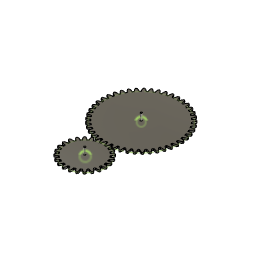
Task 5 v1 (Autodesk Fusion 360 design; units mm, degrees)
description: Spur Gear; Module: 12.700000; Num Teeth: 24; Pressure Angle: 20.000000; Backlash: 0.00 mm
description: Spur Gear; Module: 12.7; Num Teeth: 45; Pressure Angle: 20.0; Backlash: 0.00 mm
Autodesk Fusion 360 part; units mm, degrees
(part 1 of 8)
sketch "Sketch1" plane through (0, 0, 0) normal (0, 0, 1) x (1, 0, 0) in component "Spur Gear (24 teeth)"
  circle A0 centre (0, 0) radius 137.1092
  circle A1 centre (0, 0) radius 6.35
extrude "Extrude1" add sketch "Sketch1" along normal blind 12.7 makes body 1 in component "Spur Gear (24 teeth)"
sketch "Sketch2" plane through (0, 0, 0) normal (0, 0, 1) x (1, 0, 0) in component "Spur Gear (24 teeth)"
  spline S0 degree 5 poles (142.7471, -11.4951) (142.8118, -11.5003) (142.9412, -11.509) (143.1354, -11.5173) (143.3946, -11.5189) (143.7188, -11.5082) (144.0433, -11.4883) (144.3678, -11.4628) (144.6924, -11.4343) (145.0169, -11.4038) (145.3415, -11.3711) (145.666, -11.3355) (145.9905, -11.2961) (146.3148, -11.2522) (146.6391, -11.2039) (146.9633, -11.1516) (147.2873, -11.0957) (147.6112, -11.037) (147.935, -10.9757) (148.2586, -10.9121) (148.5821, -10.846) (148.9053, -10.7774) (149.2285, -10.7062) (149.5514, -10.6322) (149.8741, -10.5555) (150.1966, -10.4762) (150.5189, -10.3945) (150.8411, -10.3105) (151.1629, -10.2242) (151.4846, -10.1358) (151.806, -10.0451) (152.1272, -9.9523) (152.4482, -9.8574) (152.7689, -9.7602) (153.0893, -9.661) (153.4095, -9.5596) (153.7295, -9.4562) (154.0491, -9.3508) (154.3685, -9.2434) (154.6877, -9.1341) (155.0065, -9.0228) (155.325, -8.9096) (155.6433, -8.7946) (155.9613, -8.6776) (156.279, -8.5588) (156.5963, -8.4382) (156.9134, -8.3157) (157.2301, -8.1914) (157.5466, -8.0654) (157.8627, -7.9376) (158.1785, -7.808) (158.494, -7.6767) (158.8091, -7.5437) (159.1239, -7.409) (159.4384, -7.2727) (159.7525, -7.1346) (160.0663, -6.9949) (160.3798, -6.8535) (160.6929, -6.7105) (161.0056, -6.5659) (161.318, -6.4196) (161.63, -6.2718) (161.9417, -6.1224) (162.253, -5.9714) (162.5639, -5.8189) (162.8745, -5.6648) (163.1846, -5.5091) (163.4944, -5.352) (163.8038, -5.1933) (164.1128, -5.0331) (164.4215, -4.8714) (164.6681, -4.7409) (164.8528, -4.6423) (164.9759, -4.5763) (165.0375, -4.5432) knots 0 0 0 0 0 0 0.01428571 0.02857143 0.04285714 0.05714286 0.07142857 0.08571429 0.1 0.11428571 0.12857143 0.14285714 0.15714286 0.17142857 0.18571429 0.2 0.21428571 0.22857143 0.24285714 0.25714286 0.27142857 0.28571429 0.3 0.31428571 0.32857143 0.34285714 0.35714286 0.37142857 0.38571429 0.4 0.41428571 0.42857143 0.44285714 0.45714286 0.47142857 0.48571429 0.5 0.51428571 0.52857143 0.54285714 0.55714286 0.57142857 0.58571429 0.6 0.61428571 0.62857143 0.64285714 0.65714286 0.67142857 0.68571429 0.7 0.71428571 0.72857143 0.74285714 0.75714286 0.77142857 0.78571429 0.8 0.81428571 0.82857143 0.84285714 0.85714286 0.87142857 0.88571429 0.9 0.91428571 0.92857143 0.94285714 0.95714286 0.97142857 0.98571429 1 1 1 1 1 1
  spline S1 degree 5 poles (142.7471, 11.4951) (142.8118, 11.5003) (142.9412, 11.509) (143.1354, 11.5173) (143.3946, 11.5189) (143.7188, 11.5082) (144.0433, 11.4883) (144.3678, 11.4628) (144.6924, 11.4343) (145.0169, 11.4038) (145.3415, 11.3711) (145.666, 11.3355) (145.9905, 11.2961) (146.3148, 11.2522) (146.6391, 11.2039) (146.9633, 11.1516) (147.2873, 11.0957) (147.6112, 11.037) (147.935, 10.9757) (148.2586, 10.9121) (148.5821, 10.846) (148.9053, 10.7774) (149.2285, 10.7062) (149.5514, 10.6322) (149.8741, 10.5555) (150.1966, 10.4762) (150.5189, 10.3945) (150.8411, 10.3105) (151.1629, 10.2242) (151.4846, 10.1358) (151.806, 10.0451) (152.1272, 9.9523) (152.4482, 9.8574) (152.7689, 9.7602) (153.0893, 9.661) (153.4095, 9.5596) (153.7295, 9.4562) (154.0491, 9.3508) (154.3685, 9.2434) (154.6877, 9.1341) (155.0065, 9.0228) (155.325, 8.9096) (155.6433, 8.7946) (155.9613, 8.6776) (156.279, 8.5588) (156.5963, 8.4382) (156.9134, 8.3157) (157.2301, 8.1914) (157.5466, 8.0654) (157.8627, 7.9376) (158.1785, 7.808) (158.494, 7.6767) (158.8091, 7.5437) (159.1239, 7.409) (159.4384, 7.2727) (159.7525, 7.1346) (160.0663, 6.9949) (160.3798, 6.8535) (160.6929, 6.7105) (161.0056, 6.5659) (161.318, 6.4196) (161.63, 6.2718) (161.9417, 6.1224) (162.253, 5.9714) (162.5639, 5.8189) (162.8745, 5.6648) (163.1846, 5.5091) (163.4944, 5.352) (163.8038, 5.1933) (164.1128, 5.0331) (164.4215, 4.8714) (164.6681, 4.7409) (164.8528, 4.6423) (164.9759, 4.5763) (165.0375, 4.5432) knots 0 0 0 0 0 0 0.01428571 0.02857143 0.04285714 0.05714286 0.07142857 0.08571429 0.1 0.11428571 0.12857143 0.14285714 0.15714286 0.17142857 0.18571429 0.2 0.21428571 0.22857143 0.24285714 0.25714286 0.27142857 0.28571429 0.3 0.31428571 0.32857143 0.34285714 0.35714286 0.37142857 0.38571429 0.4 0.41428571 0.42857143 0.44285714 0.45714286 0.47142857 0.48571429 0.5 0.51428571 0.52857143 0.54285714 0.55714286 0.57142857 0.58571429 0.6 0.61428571 0.62857143 0.64285714 0.65714286 0.67142857 0.68571429 0.7 0.71428571 0.72857143 0.74285714 0.75714286 0.77142857 0.78571429 0.8 0.81428571 0.82857143 0.84285714 0.85714286 0.87142857 0.88571429 0.9 0.91428571 0.92857143 0.94285714 0.95714286 0.97142857 0.98571429 1 1 1 1 1 1
  arc A0 (165.0375, -4.5432) -> (165.0375, 4.5432) centre (0, 0) ccw
  line L0 (136.6568, -11.0055) -> (142.7471, -11.4951)
  line L1 (136.6568, 11.0055) -> (142.7471, 11.4951)
  line L2 (136.6568, -11.0055) -> (136.6568, 11.0055)
  point P0 (144.318, -11.4661)
  point P1 (145.899, -11.3066)
  point P2 (147.486, -11.0593)
  point P3 (149.0774, -10.7392)
  point P4 (150.672, -10.3543)
  point P5 (152.2688, -9.9102)
  point P6 (153.8671, -9.4106)
  point P7 (155.466, -8.8584)
  point P8 (157.065, -8.256)
  point P9 (158.6633, -7.605)
  point P10 (160.2603, -6.9071)
  point P11 (161.8554, -6.1635)
  point P12 (163.448, -5.3752)
  point P13 (144.318, 11.4661)
  point P14 (145.899, 11.3066)
  point P15 (147.486, 11.0593)
  point P16 (149.0774, 10.7392)
  point P17 (150.672, 10.3543)
  point P18 (152.2688, 9.9102)
  point P19 (153.8671, 9.4106)
  point P20 (155.466, 8.8584)
  point P21 (157.065, 8.256)
  point P22 (158.6633, 7.605)
  point P23 (160.2603, 6.9071)
  point P24 (161.8554, 6.1635)
  point P25 (163.448, 5.3752)
extrude "Extrude2" add sketch "Sketch2" along normal blind 12.7 bodies 1 in component "Spur Gear (24 teeth)"
fillet "Fillet1" radius 1.5875 2 edges at (136.6667, -11.0062, 6.35) (136.6667, 11.0062, 6.35) on bodies 1 in component "Spur Gear (24 teeth)"
pattern_circular "C-Pattern1" count 24 over 360 about axis through (0, 0, 0) along (0, 0, 1) of "Extrude2", "Fillet1" in component "Spur Gear (24 teeth)"
sketch "Sketch3" plane through (0, 0, 0) normal (0, 0, 1) x (1, 0, 0) in component "Spur Gear (24 teeth)"
  circle A0 centre (0, 0) radius 152.4 construction
sketch "Sketch1 (2)" plane through (0, 0, 0) normal (0, 0, 1) x (1, 0, 0) in component "Spur Gear (45 teeth)"
  circle A0 centre (0, 0) radius 270.4592
  circle A1 centre (0, 0) radius 6.35
extrude "Extrude1'" add sketch "Sketch1 (2)" along normal blind 12.7 separate body makes body 2 in component "Spur Gear (45 teeth)"
sketch "Sketch2 (2)" plane through (0, 0, 0) normal (0, 0, 1) x (1, 0, 0) in component "Spur Gear (45 teeth)"
  spline S0 degree 5 poles (268.1841, -13.3696) (268.2719, -13.37) (268.4476, -13.3702) (268.711, -13.3684) (269.0623, -13.3616) (269.5014, -13.3459) (269.9405, -13.3231) (270.3795, -13.2934) (270.8186, -13.2572) (271.2575, -13.215) (271.6964, -13.1674) (272.1352, -13.115) (272.5738, -13.0584) (273.0123, -12.9981) (273.4506, -12.9342) (273.8887, -12.8669) (274.3266, -12.7961) (274.7643, -12.7219) (275.2018, -12.6443) (275.6391, -12.5632) (276.0762, -12.479) (276.5131, -12.3917) (276.9498, -12.3014) (277.3862, -12.2082) (277.8224, -12.1123) (278.2583, -12.0137) (278.694, -11.9123) (279.1295, -11.8083) (279.5647, -11.7016) (279.9996, -11.5924) (280.4343, -11.4806) (280.8687, -11.3663) (281.3029, -11.2496) (281.7368, -11.1305) (282.1703, -11.009) (282.6036, -10.8852) (283.0367, -10.7592) (283.4694, -10.6308) (283.9018, -10.5002) (284.334, -10.3674) (284.7658, -10.2324) (285.1974, -10.0952) (285.6286, -9.9559) (286.0595, -9.8145) (286.4902, -9.6711) (286.9205, -9.5255) (287.3505, -9.378) (287.7801, -9.2284) (288.2095, -9.0768) (288.6385, -8.9232) (289.0672, -8.7676) (289.4956, -8.6102) (289.9236, -8.4508) (290.3513, -8.2894) (290.7786, -8.1262) (291.2056, -7.9612) (291.6323, -7.7942) (292.0586, -7.6255) (292.4846, -7.4549) (292.9102, -7.2824) (293.3355, -7.1082) (293.7604, -6.9322) (294.1849, -6.7544) (294.6091, -6.5749) (295.033, -6.3936) (295.4564, -6.2106) (295.8795, -6.0259) (296.3022, -5.8394) (296.7246, -5.6513) (297.1465, -5.4615) (297.5681, -5.27) (297.9051, -5.1155) (298.1576, -4.9988) (298.3259, -4.9207) (298.4101, -4.8816) knots 0 0 0 0 0 0 0.01428571 0.02857143 0.04285714 0.05714286 0.07142857 0.08571429 0.1 0.11428571 0.12857143 0.14285714 0.15714286 0.17142857 0.18571429 0.2 0.21428571 0.22857143 0.24285714 0.25714286 0.27142857 0.28571429 0.3 0.31428571 0.32857143 0.34285714 0.35714286 0.37142857 0.38571429 0.4 0.41428571 0.42857143 0.44285714 0.45714286 0.47142857 0.48571429 0.5 0.51428571 0.52857143 0.54285714 0.55714286 0.57142857 0.58571429 0.6 0.61428571 0.62857143 0.64285714 0.65714286 0.67142857 0.68571429 0.7 0.71428571 0.72857143 0.74285714 0.75714286 0.77142857 0.78571429 0.8 0.81428571 0.82857143 0.84285714 0.85714286 0.87142857 0.88571429 0.9 0.91428571 0.92857143 0.94285714 0.95714286 0.97142857 0.98571429 1 1 1 1 1 1
  spline S1 degree 5 poles (268.1841, 13.3696) (268.2719, 13.37) (268.4476, 13.3702) (268.711, 13.3684) (269.0623, 13.3616) (269.5014, 13.3459) (269.9405, 13.3231) (270.3795, 13.2934) (270.8186, 13.2572) (271.2575, 13.215) (271.6964, 13.1674) (272.1352, 13.115) (272.5738, 13.0584) (273.0123, 12.9981) (273.4506, 12.9342) (273.8887, 12.8669) (274.3266, 12.7961) (274.7643, 12.7219) (275.2018, 12.6443) (275.6391, 12.5632) (276.0762, 12.479) (276.5131, 12.3917) (276.9498, 12.3014) (277.3862, 12.2082) (277.8224, 12.1123) (278.2583, 12.0137) (278.694, 11.9123) (279.1295, 11.8083) (279.5647, 11.7016) (279.9996, 11.5924) (280.4343, 11.4806) (280.8687, 11.3663) (281.3029, 11.2496) (281.7368, 11.1305) (282.1703, 11.009) (282.6036, 10.8852) (283.0367, 10.7592) (283.4694, 10.6308) (283.9018, 10.5002) (284.334, 10.3674) (284.7658, 10.2324) (285.1974, 10.0952) (285.6286, 9.9559) (286.0595, 9.8145) (286.4902, 9.6711) (286.9205, 9.5255) (287.3505, 9.378) (287.7801, 9.2284) (288.2095, 9.0768) (288.6385, 8.9232) (289.0672, 8.7676) (289.4956, 8.6102) (289.9236, 8.4508) (290.3513, 8.2894) (290.7786, 8.1262) (291.2056, 7.9612) (291.6323, 7.7942) (292.0586, 7.6255) (292.4846, 7.4549) (292.9102, 7.2824) (293.3355, 7.1082) (293.7604, 6.9322) (294.1849, 6.7544) (294.6091, 6.5749) (295.033, 6.3936) (295.4564, 6.2106) (295.8795, 6.0259) (296.3022, 5.8394) (296.7246, 5.6513) (297.1465, 5.4615) (297.5681, 5.27) (297.9051, 5.1155) (298.1576, 4.9988) (298.3259, 4.9207) (298.4101, 4.8816) knots 0 0 0 0 0 0 0.01428571 0.02857143 0.04285714 0.05714286 0.07142857 0.08571429 0.1 0.11428571 0.12857143 0.14285714 0.15714286 0.17142857 0.18571429 0.2 0.21428571 0.22857143 0.24285714 0.25714286 0.27142857 0.28571429 0.3 0.31428571 0.32857143 0.34285714 0.35714286 0.37142857 0.38571429 0.4 0.41428571 0.42857143 0.44285714 0.45714286 0.47142857 0.48571429 0.5 0.51428571 0.52857143 0.54285714 0.55714286 0.57142857 0.58571429 0.6 0.61428571 0.62857143 0.64285714 0.65714286 0.67142857 0.68571429 0.7 0.71428571 0.72857143 0.74285714 0.75714286 0.77142857 0.78571429 0.8 0.81428571 0.82857143 0.84285714 0.85714286 0.87142857 0.88571429 0.9 0.91428571 0.92857143 0.94285714 0.95714286 0.97142857 0.98571429 1 1 1 1 1 1
  arc A0 (298.4101, -4.8816) -> (298.4101, 4.8816) centre (0, 0) ccw
  line L0 (268.1841, 13.3696) -> (268.1841, -13.3696)
  point P0 (270.3285, -13.2956)
  point P1 (272.48, -13.0699)
  point P2 (274.6359, -12.7432)
  point P3 (276.7948, -12.333)
  point P4 (278.9559, -11.8494)
  point P5 (281.1186, -11.2988)
  point P6 (283.2821, -10.6861)
  point P7 (285.446, -10.0146)
  point P8 (287.6098, -9.2874)
  point P9 (289.7729, -8.5066)
  point P10 (291.935, -7.6741)
  point P11 (294.0955, -6.7916)
  point P12 (296.254, -5.8603)
  point P13 (270.3285, 13.2956)
  point P14 (272.48, 13.0699)
  point P15 (274.6359, 12.7432)
  point P16 (276.7948, 12.333)
  point P17 (278.9559, 11.8494)
  point P18 (281.1186, 11.2988)
  point P19 (283.2821, 10.6861)
  point P20 (285.446, 10.0146)
  point P21 (287.6098, 9.2874)
  point P22 (289.7729, 8.5066)
  point P23 (291.935, 7.6741)
  point P24 (294.0955, 6.7916)
  point P25 (296.254, 5.8603)
extrude "Extrude2'" add sketch "Sketch2 (2)" along normal blind 12.7 bodies 2 in component "Spur Gear (45 teeth)"
fillet "Fillet1'" radius 1.5875 2 edges at (270.1315, 13.3093, 6.35) (270.1315, -13.3093, 6.35) on bodies 2 in component "Spur Gear (45 teeth)"
pattern_circular "C-Pattern1'" count 45 over 360 about axis through (0, 0, 0) along (0, 0, 1) of "Extrude2'", "Fillet1'" in component "Spur Gear (45 teeth)"
sketch "Sketch3 (2)" plane through (0, 0, 0) normal (0, 0, 1) x (1, 0, 0) in component "Spur Gear (45 teeth)"
  circle A0 centre (0, 0) radius 285.75 construction
move_body "Move1" bodies 1 to x (1, 0, 0) y (0, 1, 0) z (0, 0, 1) at (-2.1352, -2.5578, 0) in component "Spur Gear (24 teeth)"
sketch "Sketch1 (3)" plane through (0, 0, 12.7) normal (0, 0, 1) x (-1, 0, 0)
  arc A0 (-255.2626, -394.3521) -> (-256.4293, -402.6532) centre (11.949, -436.1388) ccw
  spline S0 degree 3 poles (-257.9444, -404.043) (-257.7378, -404.0351) (-257.5347, -403.987) (-257.1585, -403.8157) (-256.9889, -403.6941) (-256.733, -403.4217) (-256.6386, -403.2827) (-256.4966, -402.9803) (-256.4499, -402.8189) (-256.4293, -402.6532) knots 0 0 0 0 0.062015 0.062015 0.12403 0.12403 0.174133 0.174133 0.224236 0.224236 0.224236 0.224236
  spline S1 degree 5 poles (-257.9444, -404.043) (-257.9889, -404.0447) (-258.1217, -404.0499) (-258.3428, -404.0595) (-258.6521, -404.0751) (-259.0499, -404.0983) (-259.4915, -404.128) (-259.9332, -404.1611) (-260.3749, -404.1977) (-260.8167, -404.2378) (-261.2585, -404.2813) (-261.7004, -404.3282) (-262.1423, -404.3785) (-262.5842, -404.432) (-263.0261, -404.4887) (-263.468, -404.5483) (-263.9099, -404.6108) (-264.3517, -404.676) (-264.7935, -404.7441) (-265.2352, -404.8148) (-265.6768, -404.8882) (-266.1184, -404.9642) (-266.5599, -405.0428) (-267.0014, -405.124) (-267.4427, -405.2077) (-267.8839, -405.2939) (-268.325, -405.3824) (-268.766, -405.4733) (-269.2069, -405.5666) (-269.6477, -405.6622) (-270.0883, -405.76) (-270.5288, -405.8601) (-270.9692, -405.9625) (-271.4094, -406.067) (-271.8494, -406.1738) (-272.2893, -406.2826) (-272.7291, -406.3936) (-273.1687, -406.5067) (-273.6081, -406.6219) (-274.0473, -406.7391) (-274.4864, -406.8584) (-274.9252, -406.9796) (-275.3639, -407.1029) (-275.8024, -407.2282) (-276.2407, -407.3554) (-276.6788, -407.4845) (-277.1167, -407.6156) (-277.5544, -407.7486) (-277.9919, -407.8835) (-278.4292, -408.0203) (-278.8663, -408.1589) (-279.3031, -408.2994) (-279.7397, -408.4417) (-280.1761, -408.5858) (-280.6122, -408.7317) (-281.0481, -408.8795) (-281.4838, -409.029) (-281.9193, -409.1803) (-282.3545, -409.3333) (-282.7894, -409.4881) (-283.2241, -409.6445) (-283.6585, -409.8028) (-284.0927, -409.9627) (-284.5266, -410.1243) (-284.8736, -410.255) (-285.1336, -410.3537) (-285.307, -410.4199) (-285.3936, -410.453) knots 0.10707295 0.10707295 0.10707295 0.10707295 0.10707295 0.10707295 0.11428571 0.12857143 0.14285714 0.15714286 0.17142857 0.18571429 0.2 0.21428571 0.22857143 0.24285714 0.25714286 0.27142857 0.28571429 0.3 0.31428571 0.32857143 0.34285714 0.35714286 0.37142857 0.38571429 0.4 0.41428571 0.42857143 0.44285714 0.45714286 0.47142857 0.48571429 0.5 0.51428571 0.52857143 0.54285714 0.55714286 0.57142857 0.58571429 0.6 0.61428571 0.62857143 0.64285714 0.65714286 0.67142857 0.68571429 0.7 0.71428571 0.72857143 0.74285714 0.75714286 0.77142857 0.78571429 0.8 0.81428571 0.82857143 0.84285714 0.85714286 0.87142857 0.88571429 0.9 0.91428571 0.92857143 0.94285714 0.95714286 0.97142857 0.98571429 1 1 1 1 1 1
  arc A1 (-285.3936, -410.453) -> (-286.0747, -420.1924) centre (11.949, -436.1388) ccw
  spline S2 degree 5 poles (-286.0747, -420.1924) (-285.9935, -420.2373) (-285.831, -420.327) (-285.5872, -420.461) (-285.2619, -420.6386) (-284.8547, -420.8591) (-284.447, -421.0778) (-284.0388, -421.295) (-283.6301, -421.5104) (-283.2209, -421.7242) (-282.8113, -421.9363) (-282.4011, -422.1468) (-281.9905, -422.3554) (-281.5794, -422.5624) (-281.1678, -422.7676) (-280.7557, -422.9711) (-280.3431, -423.1728) (-279.9301, -423.3727) (-279.5166, -423.5708) (-279.1026, -423.7671) (-278.6882, -423.9615) (-278.2732, -424.1541) (-277.8578, -424.3449) (-277.442, -424.5338) (-277.0256, -424.7207) (-276.6088, -424.9058) (-276.1916, -425.0889) (-275.7738, -425.2701) (-275.3557, -425.4493) (-274.937, -425.6265) (-274.5179, -425.8017) (-274.0983, -425.9749) (-273.6783, -426.146) (-273.2579, -426.315) (-272.8369, -426.482) (-272.4155, -426.6468) (-271.9937, -426.8094) (-271.5714, -426.9698) (-271.1487, -427.1281) (-270.7255, -427.2841) (-270.3019, -427.4378) (-269.8779, -427.5892) (-269.4534, -427.7383) (-269.0284, -427.885) (-268.603, -428.0293) (-268.1772, -428.1711) (-267.751, -428.3104) (-267.3243, -428.4472) (-266.8971, -428.5813) (-266.4695, -428.7128) (-266.0415, -428.8417) (-265.6131, -428.9678) (-265.1842, -429.0911) (-264.7549, -429.2117) (-264.3252, -429.3293) (-263.895, -429.4438) (-263.4644, -429.5551) (-263.0334, -429.6631) (-262.6019, -429.7677) (-262.17, -429.8688) (-261.7377, -429.9665) (-261.3049, -430.0608) (-260.8718, -430.1516) (-260.4811, -430.23) (-260.1769, -430.2885) (-259.9593, -430.3288) (-259.8285, -430.3524) (-259.7847, -430.3603) knots -1 -1 -1 -1 -1 -1 -0.98571429 -0.97142857 -0.95714286 -0.94285714 -0.92857143 -0.91428571 -0.9 -0.88571429 -0.87142857 -0.85714286 -0.84285714 -0.82857143 -0.81428571 -0.8 -0.78571429 -0.77142857 -0.75714286 -0.74285714 -0.72857143 -0.71428571 -0.7 -0.68571429 -0.67142857 -0.65714286 -0.64285714 -0.62857143 -0.61428571 -0.6 -0.58571429 -0.57142857 -0.55714286 -0.54285714 -0.52857143 -0.51428571 -0.5 -0.48571429 -0.47142857 -0.45714286 -0.44285714 -0.42857143 -0.41428571 -0.4 -0.38571429 -0.37142857 -0.35714286 -0.34285714 -0.32857143 -0.31428571 -0.3 -0.28571429 -0.27142857 -0.25714286 -0.24285714 -0.22857143 -0.21428571 -0.2 -0.18571429 -0.17142857 -0.15714286 -0.14285714 -0.12857143 -0.11428571 -0.10707295 -0.10707295 -0.10707295 -0.10707295 -0.10707295 -0.10707295
  spline S3 degree 3 poles (-258.4777, -431.9474) (-258.4745, -431.7408) (-258.5117, -431.5354) (-258.6627, -431.1505) (-258.7751, -430.9747) (-259.0335, -430.7047) (-259.1672, -430.603) (-259.4616, -430.445) (-259.6203, -430.3898) (-259.7847, -430.3603) knots 0 0 0 0 0.062015 0.062015 0.12403 0.12403 0.174133 0.174133 0.224236 0.224236 0.224236 0.224236
  arc A2 (-258.4777, -431.9474) -> (-258.4777, -440.3301) centre (11.949, -436.1388) ccw
  spline S4 degree 3 poles (-259.7847, -441.9172) (-259.5812, -441.8807) (-259.3868, -441.8048) (-259.0381, -441.5828) (-258.887, -441.4388) (-258.6716, -441.1334) (-258.5974, -440.9826) (-258.4989, -440.6634) (-258.4751, -440.4971) (-258.4777, -440.3301) knots 0 0 0 0 0.062015 0.062015 0.12403 0.12403 0.174133 0.174133 0.224236 0.224236 0.224236 0.224236
  spline S5 degree 5 poles (-259.7847, -441.9172) (-259.8285, -441.9251) (-259.9593, -441.9488) (-260.1769, -441.9891) (-260.4811, -442.0475) (-260.8718, -442.1259) (-261.3049, -442.2167) (-261.7377, -442.311) (-262.17, -442.4087) (-262.6019, -442.5099) (-263.0334, -442.6144) (-263.4644, -442.7224) (-263.895, -442.8337) (-264.3252, -442.9483) (-264.7549, -443.0659) (-265.1842, -443.1864) (-265.6131, -443.3098) (-266.0415, -443.4359) (-266.4695, -443.5647) (-266.8971, -443.6962) (-267.3243, -443.8303) (-267.751, -443.9671) (-268.1772, -444.1064) (-268.603, -444.2482) (-269.0284, -444.3926) (-269.4534, -444.5393) (-269.8779, -444.6883) (-270.3019, -444.8398) (-270.7255, -444.9935) (-271.1487, -445.1495) (-271.5714, -445.3077) (-271.9937, -445.4681) (-272.4155, -445.6308) (-272.8369, -445.7956) (-273.2579, -445.9625) (-273.6783, -446.1315) (-274.0983, -446.3026) (-274.5179, -446.4758) (-274.937, -446.651) (-275.3557, -446.8282) (-275.7738, -447.0074) (-276.1916, -447.1886) (-276.6088, -447.3717) (-277.0256, -447.5568) (-277.442, -447.7438) (-277.8578, -447.9326) (-278.2732, -448.1234) (-278.6882, -448.316) (-279.1026, -448.5105) (-279.5166, -448.7068) (-279.9301, -448.9049) (-280.3431, -449.1048) (-280.7557, -449.3064) (-281.1678, -449.5099) (-281.5794, -449.7151) (-281.9905, -449.9221) (-282.4011, -450.1308) (-282.8113, -450.3412) (-283.2209, -450.5533) (-283.6301, -450.7671) (-284.0388, -450.9825) (-284.447, -451.1997) (-284.8547, -451.4185) (-285.2619, -451.6389) (-285.5872, -451.8166) (-285.831, -451.9506) (-285.9935, -452.0402) (-286.0747, -452.0851) knots 0.10707295 0.10707295 0.10707295 0.10707295 0.10707295 0.10707295 0.11428571 0.12857143 0.14285714 0.15714286 0.17142857 0.18571429 0.2 0.21428571 0.22857143 0.24285714 0.25714286 0.27142857 0.28571429 0.3 0.31428571 0.32857143 0.34285714 0.35714286 0.37142857 0.38571429 0.4 0.41428571 0.42857143 0.44285714 0.45714286 0.47142857 0.48571429 0.5 0.51428571 0.52857143 0.54285714 0.55714286 0.57142857 0.58571429 0.6 0.61428571 0.62857143 0.64285714 0.65714286 0.67142857 0.68571429 0.7 0.71428571 0.72857143 0.74285714 0.75714286 0.77142857 0.78571429 0.8 0.81428571 0.82857143 0.84285714 0.85714286 0.87142857 0.88571429 0.9 0.91428571 0.92857143 0.94285714 0.95714286 0.97142857 0.98571429 1 1 1 1 1 1
  arc A3 (-286.0747, -452.0851) -> (-285.3936, -461.8245) centre (11.949, -436.1388) ccw
  spline S6 degree 5 poles (-285.3936, -461.8245) (-285.307, -461.8576) (-285.1336, -461.9238) (-284.8736, -462.0226) (-284.5266, -462.1532) (-284.0927, -462.3148) (-283.6585, -462.4748) (-283.2241, -462.633) (-282.7894, -462.7895) (-282.3545, -462.9442) (-281.9193, -463.0973) (-281.4838, -463.2485) (-281.0481, -463.3981) (-280.6122, -463.5458) (-280.1761, -463.6917) (-279.7397, -463.8358) (-279.3031, -463.9782) (-278.8663, -464.1186) (-278.4292, -464.2573) (-277.9919, -464.394) (-277.5544, -464.5289) (-277.1167, -464.6619) (-276.6788, -464.793) (-276.2407, -464.9221) (-275.8024, -465.0494) (-275.3639, -465.1746) (-274.9252, -465.2979) (-274.4864, -465.4192) (-274.0473, -465.5384) (-273.6081, -465.6557) (-273.1687, -465.7708) (-272.7291, -465.8839) (-272.2893, -465.9949) (-271.8494, -466.1038) (-271.4094, -466.2105) (-270.9692, -466.315) (-270.5288, -466.4174) (-270.0883, -466.5175) (-269.6477, -466.6154) (-269.2069, -466.7109) (-268.766, -466.8042) (-268.325, -466.8951) (-267.8839, -466.9837) (-267.4427, -467.0698) (-267.0014, -467.1535) (-266.5599, -467.2347) (-266.1184, -467.3133) (-265.6768, -467.3894) (-265.2352, -467.4628) (-264.7935, -467.5335) (-264.3517, -467.6015) (-263.9099, -467.6667) (-263.468, -467.7292) (-263.0261, -467.7888) (-262.5842, -467.8455) (-262.1423, -467.899) (-261.7004, -467.9493) (-261.2585, -467.9963) (-260.8167, -468.0398) (-260.3749, -468.0798) (-259.9332, -468.1164) (-259.4915, -468.1496) (-259.0499, -468.1792) (-258.6521, -468.2025) (-258.3428, -468.218) (-258.1217, -468.2276) (-257.9889, -468.2329) (-257.9444, -468.2345) knots -1 -1 -1 -1 -1 -1 -0.98571429 -0.97142857 -0.95714286 -0.94285714 -0.92857143 -0.91428571 -0.9 -0.88571429 -0.87142857 -0.85714286 -0.84285714 -0.82857143 -0.81428571 -0.8 -0.78571429 -0.77142857 -0.75714286 -0.74285714 -0.72857143 -0.71428571 -0.7 -0.68571429 -0.67142857 -0.65714286 -0.64285714 -0.62857143 -0.61428571 -0.6 -0.58571429 -0.57142857 -0.55714286 -0.54285714 -0.52857143 -0.51428571 -0.5 -0.48571429 -0.47142857 -0.45714286 -0.44285714 -0.42857143 -0.41428571 -0.4 -0.38571429 -0.37142857 -0.35714286 -0.34285714 -0.32857143 -0.31428571 -0.3 -0.28571429 -0.27142857 -0.25714286 -0.24285714 -0.22857143 -0.21428571 -0.2 -0.18571429 -0.17142857 -0.15714286 -0.14285714 -0.12857143 -0.11428571 -0.10707295 -0.10707295 -0.10707295 -0.10707295 -0.10707295 -0.10707295
  spline S7 degree 3 poles (-256.4293, -469.6244) (-256.4549, -469.4192) (-256.5203, -469.2211) (-256.7234, -468.861) (-256.8591, -468.7025) (-257.1526, -468.471) (-257.2992, -468.3889) (-257.6126, -468.2735) (-257.7775, -468.2409) (-257.9444, -468.2345) knots 0 0 0 0 0.062015 0.062015 0.12403 0.12403 0.174133 0.174133 0.224236 0.224236 0.224236 0.224236
  arc A4 (-256.4293, -469.6244) -> (-255.2626, -477.9254) centre (11.949, -436.1388) ccw
  spline S8 degree 3 poles (-256.336, -479.679) (-256.1396, -479.6145) (-255.9576, -479.5123) (-255.6432, -479.2439) (-255.5137, -479.0803) (-255.3428, -478.7479) (-255.2904, -478.5882) (-255.2372, -478.2585) (-255.2368, -478.0904) (-255.2626, -477.9254) knots 0 0 0 0 0.062015 0.062015 0.12403 0.12403 0.174133 0.174133 0.224236 0.224236 0.224236 0.224236
  spline S9 degree 5 poles (-256.336, -479.679) (-256.3783, -479.6929) (-256.5045, -479.7345) (-256.7143, -479.8047) (-257.0075, -479.905) (-257.3834, -480.037) (-257.7998, -480.1872) (-258.2152, -480.3408) (-258.6297, -480.4977) (-259.0433, -480.658) (-259.456, -480.8216) (-259.8679, -480.9885) (-260.2788, -481.1586) (-260.6888, -481.3319) (-261.098, -481.5082) (-261.5063, -481.6873) (-261.9139, -481.8691) (-262.3206, -482.0537) (-262.7265, -482.2408) (-263.1316, -482.4305) (-263.5359, -482.6228) (-263.9394, -482.8176) (-264.3422, -483.0149) (-264.7441, -483.2146) (-265.1453, -483.4167) (-265.5457, -483.6212) (-265.9453, -483.8279) (-266.3441, -484.0368) (-266.7422, -484.248) (-267.1396, -484.4613) (-267.5362, -484.6769) (-267.932, -484.8945) (-268.3271, -485.1143) (-268.7214, -485.3361) (-269.115, -485.56) (-269.5079, -485.7859) (-269.9, -486.0138) (-270.2914, -486.2437) (-270.682, -486.4755) (-271.0719, -486.7093) (-271.4611, -486.9449) (-271.8496, -487.1825) (-272.2373, -487.4219) (-272.6243, -487.6632) (-273.0105, -487.9063) (-273.3961, -488.1512) (-273.7809, -488.3979) (-274.165, -488.6464) (-274.5483, -488.8966) (-274.9309, -489.1486) (-275.3129, -489.4023) (-275.6941, -489.6578) (-276.0745, -489.9149) (-276.4543, -490.1737) (-276.8333, -490.4342) (-277.2116, -490.6964) (-277.5892, -490.9602) (-277.9661, -491.2257) (-278.3422, -491.4927) (-278.7177, -491.7614) (-279.0924, -492.0316) (-279.4664, -492.3035) (-279.8397, -492.5769) (-280.2122, -492.8518) (-280.5097, -493.073) (-280.7325, -493.2396) (-280.8809, -493.351) (-280.955, -493.4068) knots 0.10707295 0.10707295 0.10707295 0.10707295 0.10707295 0.10707295 0.11428571 0.12857143 0.14285714 0.15714286 0.17142857 0.18571429 0.2 0.21428571 0.22857143 0.24285714 0.25714286 0.27142857 0.28571429 0.3 0.31428571 0.32857143 0.34285714 0.35714286 0.37142857 0.38571429 0.4 0.41428571 0.42857143 0.44285714 0.45714286 0.47142857 0.48571429 0.5 0.51428571 0.52857143 0.54285714 0.55714286 0.57142857 0.58571429 0.6 0.61428571 0.62857143 0.64285714 0.65714286 0.67142857 0.68571429 0.7 0.71428571 0.72857143 0.74285714 0.75714286 0.77142857 0.78571429 0.8 0.81428571 0.82857143 0.84285714 0.85714286 0.87142857 0.88571429 0.9 0.91428571 0.92857143 0.94285714 0.95714286 0.97142857 0.98571429 1 1 1 1 1 1
  arc A5 (-280.955, -493.4068) -> (-278.9252, -502.9566) centre (11.949, -436.1388) ccw
  spline S10 degree 5 poles (-278.9252, -502.9566) (-278.8347, -502.9774) (-278.6539, -503.0188) (-278.3826, -503.0804) (-278.0208, -503.1615) (-277.5686, -503.2611) (-277.1164, -503.3591) (-276.6642, -503.4553) (-276.212, -503.5498) (-275.7597, -503.6425) (-275.3075, -503.7335) (-274.8552, -503.8227) (-274.403, -503.9101) (-273.9507, -503.9957) (-273.4985, -504.0795) (-273.0463, -504.1615) (-272.5941, -504.2417) (-272.142, -504.32) (-271.6899, -504.3964) (-271.2379, -504.471) (-270.7859, -504.5437) (-270.3339, -504.6145) (-269.882, -504.6834) (-269.4302, -504.7503) (-268.9785, -504.8153) (-268.5268, -504.8783) (-268.0752, -504.9393) (-267.6238, -504.9983) (-267.1724, -505.0553) (-266.7211, -505.1103) (-266.2699, -505.1632) (-265.8189, -505.214) (-265.368, -505.2627) (-264.9172, -505.3093) (-264.4666, -505.3537) (-264.0161, -505.396) (-263.5658, -505.436) (-263.1156, -505.4739) (-262.6657, -505.5094) (-262.2159, -505.5427) (-261.7663, -505.5737) (-261.317, -505.6024) (-260.8678, -505.6287) (-260.4189, -505.6526) (-259.9702, -505.674) (-259.5218, -505.693) (-259.0736, -505.7094) (-258.6258, -505.7233) (-258.1782, -505.7345) (-257.7309, -505.743) (-257.284, -505.7489) (-256.8374, -505.752) (-256.3911, -505.7524) (-255.9453, -505.75) (-255.4997, -505.7445) (-255.0547, -505.7361) (-254.6101, -505.7244) (-254.166, -505.7094) (-253.7224, -505.691) (-253.2794, -505.6691) (-252.8368, -505.6439) (-252.3948, -505.6153) (-251.9534, -505.5831) (-251.5563, -505.5508) (-251.2477, -505.5231) (-251.0275, -505.5019) (-250.8953, -505.4886) (-250.8509, -505.4841) knots -1 -1 -1 -1 -1 -1 -0.98571429 -0.97142857 -0.95714286 -0.94285714 -0.92857143 -0.91428571 -0.9 -0.88571429 -0.87142857 -0.85714286 -0.84285714 -0.82857143 -0.81428571 -0.8 -0.78571429 -0.77142857 -0.75714286 -0.74285714 -0.72857143 -0.71428571 -0.7 -0.68571429 -0.67142857 -0.65714286 -0.64285714 -0.62857143 -0.61428571 -0.6 -0.58571429 -0.57142857 -0.55714286 -0.54285714 -0.52857143 -0.51428571 -0.5 -0.48571429 -0.47142857 -0.45714286 -0.44285714 -0.42857143 -0.41428571 -0.4 -0.38571429 -0.37142857 -0.35714286 -0.34285714 -0.32857143 -0.31428571 -0.3 -0.28571429 -0.27142857 -0.25714286 -0.24285714 -0.22857143 -0.21428571 -0.2 -0.18571429 -0.17142857 -0.15714286 -0.14285714 -0.12857143 -0.11428571 -0.10707295 -0.10707295 -0.10707295 -0.10707295 -0.10707295 -0.10707295
  spline S11 degree 3 poles (-249.1571, -506.6495) (-249.211, -506.4499) (-249.3034, -506.2628) (-249.5546, -505.9345) (-249.7111, -505.7964) (-250.0339, -505.6081) (-250.1905, -505.5472) (-250.517, -505.4765) (-250.6848, -505.4671) (-250.8509, -505.4841) knots 0 0 0 0 0.062015 0.062015 0.12403 0.12403 0.174133 0.174133 0.224236 0.224236 0.224236 0.224236
  arc A6 (-249.1571, -506.6495) -> (-246.8466, -514.7074) centre (11.949, -436.1388) ccw
  spline S12 degree 3 poles (-247.6654, -516.5933) (-247.4799, -516.5022) (-247.3139, -516.3756) (-247.0399, -516.066) (-246.9344, -515.886) (-246.8115, -515.5331) (-246.7818, -515.3677) (-246.775, -515.0337) (-246.798, -514.8672) (-246.8466, -514.7074) knots 0 0 0 0 0.062015 0.062015 0.12403 0.12403 0.174133 0.174133 0.224236 0.224236 0.224236 0.224236
  spline S13 degree 5 poles (-247.6654, -516.5933) (-247.7054, -516.613) (-247.8246, -516.6718) (-248.0226, -516.7705) (-248.2989, -516.9105) (-248.6529, -517.0936) (-249.0442, -517.3002) (-249.4342, -517.5102) (-249.8229, -517.7233) (-250.2102, -517.9395) (-250.5961, -518.159) (-250.9807, -518.3816) (-251.3639, -518.6073) (-251.7458, -518.836) (-252.1265, -519.0675) (-252.506, -519.3017) (-252.8842, -519.5384) (-253.2613, -519.7778) (-253.6372, -520.0196) (-254.012, -520.2638) (-254.3856, -520.5105) (-254.7581, -520.7596) (-255.1294, -521.011) (-255.4997, -521.2647) (-255.8688, -521.5207) (-256.2368, -521.7788) (-256.6038, -522.0392) (-256.9697, -522.3016) (-257.3345, -522.5661) (-257.6983, -522.8327) (-258.061, -523.1013) (-258.4227, -523.3719) (-258.7834, -523.6445) (-259.143, -523.9191) (-259.5016, -524.1956) (-259.8592, -524.474) (-260.2158, -524.7542) (-260.5714, -525.0363) (-260.926, -525.3203) (-261.2796, -525.606) (-261.6321, -525.8935) (-261.9837, -526.1828) (-262.3344, -526.4739) (-262.684, -526.7667) (-263.0327, -527.0612) (-263.3804, -527.3574) (-263.7271, -527.6552) (-264.0729, -527.9547) (-264.4177, -528.2559) (-264.7615, -528.5587) (-265.1044, -528.8631) (-265.4463, -529.1691) (-265.7873, -529.4767) (-266.1273, -529.7859) (-266.4664, -530.0966) (-266.8046, -530.4088) (-267.1418, -530.7226) (-267.478, -531.0379) (-267.8134, -531.3547) (-268.1477, -531.673) (-268.4812, -531.9928) (-268.8137, -532.314) (-269.1453, -532.6367) (-269.476, -532.9609) (-269.7398, -533.2213) (-269.9372, -533.4173) (-270.0687, -533.5483) (-270.1343, -533.6138) knots 0.10707295 0.10707295 0.10707295 0.10707295 0.10707295 0.10707295 0.11428571 0.12857143 0.14285714 0.15714286 0.17142857 0.18571429 0.2 0.21428571 0.22857143 0.24285714 0.25714286 0.27142857 0.28571429 0.3 0.31428571 0.32857143 0.34285714 0.35714286 0.37142857 0.38571429 0.4 0.41428571 0.42857143 0.44285714 0.45714286 0.47142857 0.48571429 0.5 0.51428571 0.52857143 0.54285714 0.55714286 0.57142857 0.58571429 0.6 0.61428571 0.62857143 0.64285714 0.65714286 0.67142857 0.68571429 0.7 0.71428571 0.72857143 0.74285714 0.75714286 0.77142857 0.78571429 0.8 0.81428571 0.82857143 0.84285714 0.85714286 0.87142857 0.88571429 0.9 0.91428571 0.92857143 0.94285714 0.95714286 0.97142857 0.98571429 1 1 1 1 1 1
  arc A7 (-270.1343, -533.6138) -> (-266.7951, -542.7882) centre (11.949, -436.1388) ccw
  spline S14 degree 5 poles (-266.7951, -542.7882) (-266.7027, -542.7962) (-266.5178, -542.812) (-266.2406, -542.8353) (-265.8711, -542.8652) (-265.4094, -542.901) (-264.948, -542.935) (-264.4868, -542.9674) (-264.0258, -542.998) (-263.5651, -543.0269) (-263.1045, -543.054) (-262.6443, -543.0794) (-262.1843, -543.103) (-261.7245, -543.1249) (-261.265, -543.1449) (-260.8058, -543.1632) (-260.3469, -543.1797) (-259.8883, -543.1943) (-259.4299, -543.2071) (-258.9719, -543.218) (-258.5142, -543.2271) (-258.0568, -543.2343) (-257.5997, -543.2396) (-257.143, -543.243) (-256.6866, -543.2445) (-256.2306, -543.244) (-255.7749, -543.2416) (-255.3196, -543.2372) (-254.8647, -543.2308) (-254.4101, -543.2224) (-253.956, -543.212) (-253.5023, -543.1995) (-253.049, -543.185) (-252.5961, -543.1684) (-252.1437, -543.1497) (-251.6917, -543.1289) (-251.2402, -543.1059) (-250.7891, -543.0807) (-250.3386, -543.0533) (-249.8886, -543.0237) (-249.4391, -542.9918) (-248.9901, -542.9576) (-248.5416, -542.9212) (-248.0938, -542.8824) (-247.6465, -542.8412) (-247.1998, -542.7975) (-246.7537, -542.7514) (-246.3083, -542.7028) (-245.8635, -542.6516) (-245.4194, -542.5979) (-244.976, -542.5415) (-244.5333, -542.4824) (-244.0913, -542.4207) (-243.6501, -542.3562) (-243.2097, -542.2888) (-242.7701, -542.2185) (-242.3315, -542.145) (-241.8938, -542.0684) (-241.4571, -541.9884) (-241.0214, -541.9051) (-240.5867, -541.8186) (-240.153, -541.7287) (-239.7204, -541.6354) (-239.3316, -541.5481) (-239.0299, -541.4778) (-238.8147, -541.4261) (-238.6857, -541.3946) (-238.6424, -541.3839) knots -1 -1 -1 -1 -1 -1 -0.98571429 -0.97142857 -0.95714286 -0.94285714 -0.92857143 -0.91428571 -0.9 -0.88571429 -0.87142857 -0.85714286 -0.84285714 -0.82857143 -0.81428571 -0.8 -0.78571429 -0.77142857 -0.75714286 -0.74285714 -0.72857143 -0.71428571 -0.7 -0.68571429 -0.67142857 -0.65714286 -0.64285714 -0.62857143 -0.61428571 -0.6 -0.58571429 -0.57142857 -0.55714286 -0.54285714 -0.52857143 -0.51428571 -0.5 -0.48571429 -0.47142857 -0.45714286 -0.44285714 -0.42857143 -0.41428571 -0.4 -0.38571429 -0.37142857 -0.35714286 -0.34285714 -0.32857143 -0.31428571 -0.3 -0.28571429 -0.27142857 -0.25714286 -0.24285714 -0.22857143 -0.21428571 -0.2 -0.18571429 -0.17142857 -0.15714286 -0.14285714 -0.12857143 -0.11428571 -0.10707295 -0.10707295 -0.10707295 -0.10707295 -0.10707295 -0.10707295
  spline S15 degree 3 poles (-236.8029, -542.3023) (-236.884, -542.1121) (-237.0015, -541.9397) (-237.296, -541.6495) (-237.4702, -541.5346) (-237.816, -541.393) (-237.9796, -541.3545) (-238.3127, -541.3299) (-238.4802, -541.344) (-238.6424, -541.3839) knots 0 0 0 0 0.062015 0.062015 0.12403 0.12403 0.174133 0.174133 0.224236 0.224236 0.224236 0.224236
  arc A8 (-236.8029, -542.3023) -> (-233.3933, -549.9602) centre (11.949, -436.1388) ccw
  spline S16 degree 3 poles (-233.9417, -551.9417) (-233.7707, -551.8256) (-233.624, -551.6772) (-233.3957, -551.3325) (-233.3163, -551.1395) (-233.2437, -550.7729) (-233.2373, -550.605) (-233.2771, -550.2733) (-233.323, -550.1117) (-233.3933, -549.9602) knots 0 0 0 0 0.062015 0.062015 0.12403 0.12403 0.174133 0.174133 0.224236 0.224236 0.224236 0.224236
  spline S17 degree 5 poles (-233.9417, -551.9417) (-233.9786, -551.9667) (-234.0884, -552.0415) (-234.2708, -552.1668) (-234.525, -552.344) (-234.85, -552.5745) (-235.2088, -552.8336) (-235.5658, -553.0958) (-235.921, -553.3609) (-236.2744, -553.629) (-236.626, -553.9) (-236.9759, -554.174) (-237.324, -554.4508) (-237.6704, -554.7304) (-238.0151, -555.0126) (-238.3583, -555.2973) (-238.6999, -555.5845) (-239.04, -555.8739) (-239.3786, -556.1657) (-239.7157, -556.4598) (-240.0514, -556.756) (-240.3856, -557.0545) (-240.7183, -557.3552) (-241.0496, -557.6579) (-241.3795, -557.9628) (-241.7081, -558.2697) (-242.0352, -558.5785) (-242.361, -558.8893) (-242.6855, -559.202) (-243.0087, -559.5167) (-243.3305, -559.8331) (-243.651, -560.1515) (-243.9702, -560.4716) (-244.2881, -560.7936) (-244.6048, -561.1173) (-244.9201, -561.4427) (-245.2342, -561.7699) (-245.5471, -562.0987) (-245.8587, -562.4292) (-246.1691, -562.7614) (-246.4782, -563.0952) (-246.7861, -563.4306) (-247.0928, -563.7676) (-247.3983, -564.1062) (-247.7026, -564.4464) (-248.0057, -564.7881) (-248.3076, -565.1313) (-248.6083, -565.476) (-248.9079, -565.8222) (-249.2062, -566.1699) (-249.5034, -566.5191) (-249.7994, -566.8697) (-250.0943, -567.2218) (-250.388, -567.5752) (-250.6805, -567.9301) (-250.9719, -568.2864) (-251.2621, -568.6441) (-251.5513, -569.0031) (-251.8392, -569.3635) (-252.1261, -569.7252) (-252.4118, -570.0883) (-252.6964, -570.4527) (-252.9798, -570.8184) (-253.2622, -571.1854) (-253.4871, -571.48) (-253.6554, -571.7016) (-253.7673, -571.8496) (-253.8232, -571.9236) knots 0.10707295 0.10707295 0.10707295 0.10707295 0.10707295 0.10707295 0.11428571 0.12857143 0.14285714 0.15714286 0.17142857 0.18571429 0.2 0.21428571 0.22857143 0.24285714 0.25714286 0.27142857 0.28571429 0.3 0.31428571 0.32857143 0.34285714 0.35714286 0.37142857 0.38571429 0.4 0.41428571 0.42857143 0.44285714 0.45714286 0.47142857 0.48571429 0.5 0.51428571 0.52857143 0.54285714 0.55714286 0.57142857 0.58571429 0.6 0.61428571 0.62857143 0.64285714 0.65714286 0.67142857 0.68571429 0.7 0.71428571 0.72857143 0.74285714 0.75714286 0.77142857 0.78571429 0.8 0.81428571 0.82857143 0.84285714 0.85714286 0.87142857 0.88571429 0.9 0.91428571 0.92857143 0.94285714 0.95714286 0.97142857 0.98571429 1 1 1 1 1 1
  arc A9 (-253.8232, -571.9236) -> (-249.2397, -580.544) centre (11.949, -436.1388) ccw
  spline S18 degree 5 poles (-249.2397, -580.544) (-249.147, -580.539) (-248.9618, -580.529) (-248.684, -580.5134) (-248.3139, -580.4917) (-247.8518, -580.4628) (-247.3901, -580.4323) (-246.9289, -580.4001) (-246.4681, -580.3663) (-246.0078, -580.3308) (-245.548, -580.2936) (-245.0887, -580.2547) (-244.6299, -580.214) (-244.1715, -580.1717) (-243.7137, -580.1276) (-243.2565, -580.0818) (-242.7997, -580.0342) (-242.3435, -579.9849) (-241.8879, -579.9337) (-241.4328, -579.8808) (-240.9782, -579.8261) (-240.5243, -579.7696) (-240.0709, -579.7112) (-239.6182, -579.651) (-239.166, -579.589) (-238.7145, -579.525) (-238.2636, -579.4592) (-237.8133, -579.3915) (-237.3637, -579.3219) (-236.9148, -579.2503) (-236.4665, -579.1768) (-236.0189, -579.1013) (-235.5721, -579.0239) (-235.1259, -578.9444) (-234.6805, -578.8629) (-234.2358, -578.7793) (-233.7919, -578.6937) (-233.3488, -578.606) (-232.9064, -578.5162) (-232.4649, -578.4242) (-232.0242, -578.3301) (-231.5843, -578.2338) (-231.1453, -578.1353) (-230.7072, -578.0345) (-230.27, -577.9315) (-229.8337, -577.8261) (-229.3984, -577.7184) (-228.9641, -577.6082) (-228.5307, -577.4956) (-228.0985, -577.3806) (-227.6672, -577.263) (-227.2371, -577.1429) (-226.808, -577.0203) (-226.38, -576.895) (-225.9533, -576.767) (-225.5278, -576.6362) (-225.1036, -576.5024) (-224.6809, -576.3656) (-224.2596, -576.2256) (-223.8397, -576.0825) (-223.4213, -575.9363) (-223.0043, -575.7869) (-222.5888, -575.6343) (-222.216, -575.4938) (-221.927, -575.3822) (-221.7211, -575.3011) (-221.5977, -575.2518) (-221.5563, -575.2352) knots -1 -1 -1 -1 -1 -1 -0.98571429 -0.97142857 -0.95714286 -0.94285714 -0.92857143 -0.91428571 -0.9 -0.88571429 -0.87142857 -0.85714286 -0.84285714 -0.82857143 -0.81428571 -0.8 -0.78571429 -0.77142857 -0.75714286 -0.74285714 -0.72857143 -0.71428571 -0.7 -0.68571429 -0.67142857 -0.65714286 -0.64285714 -0.62857143 -0.61428571 -0.6 -0.58571429 -0.57142857 -0.55714286 -0.54285714 -0.52857143 -0.51428571 -0.5 -0.48571429 -0.47142857 -0.45714286 -0.44285714 -0.42857143 -0.41428571 -0.4 -0.38571429 -0.37142857 -0.35714286 -0.34285714 -0.32857143 -0.31428571 -0.3 -0.28571429 -0.27142857 -0.25714286 -0.24285714 -0.22857143 -0.21428571 -0.2 -0.18571429 -0.17142857 -0.15714286 -0.14285714 -0.12857143 -0.11428571 -0.10707295 -0.10707295 -0.10707295 -0.10707295 -0.10707295 -0.10707295
  spline S19 degree 3 poles (-219.6069, -575.8887) (-219.7137, -575.7117) (-219.8541, -575.5572) (-220.1861, -575.3109) (-220.3746, -575.2213) (-220.7368, -575.1292) (-220.9041, -575.1139) (-221.2374, -575.1359) (-221.4013, -575.1732) (-221.5563, -575.2352) knots 0 0 0 0 0.062015 0.062015 0.12403 0.12403 0.174133 0.174133 0.224236 0.224236 0.224236 0.224236
  arc A10 (-219.6069, -575.8887) -> (-215.1648, -582.9975) centre (11.949, -436.1388) ccw
  spline S20 degree 3 poles (-215.4321, -585.0361) (-215.2789, -584.8973) (-215.1543, -584.7299) (-214.9762, -584.3568) (-214.9244, -584.1547) (-214.9035, -583.7815) (-214.9206, -583.6143) (-215.0061, -583.2915) (-215.0741, -583.1378) (-215.1648, -582.9975) knots 0 0 0 0 0.062015 0.062015 0.12403 0.12403 0.174133 0.174133 0.224236 0.224236 0.224236 0.224236
  spline S21 degree 5 poles (-215.4321, -585.0361) (-215.4651, -585.066) (-215.5635, -585.1554) (-215.7266, -585.3048) (-215.9536, -585.5156) (-216.2434, -585.7891) (-216.5627, -586.0957) (-216.8797, -586.405) (-217.1945, -586.7169) (-217.5072, -587.0316) (-217.8177, -587.3489) (-218.126, -587.6689) (-218.4322, -587.9915) (-218.7363, -588.3166) (-219.0384, -588.644) (-219.3386, -588.9737) (-219.637, -589.3056) (-219.9335, -589.6396) (-220.2282, -589.9757) (-220.5211, -590.3138) (-220.8122, -590.6539) (-221.1016, -590.996) (-221.3893, -591.34) (-221.6752, -591.6859) (-221.9595, -592.0337) (-222.2422, -592.3833) (-222.5232, -592.7347) (-222.8025, -593.0878) (-223.0803, -593.4427) (-223.3565, -593.7992) (-223.6312, -594.1574) (-223.9043, -594.5172) (-224.1758, -594.8787) (-224.4458, -595.2417) (-224.7143, -595.6064) (-224.9814, -595.9725) (-225.2469, -596.3402) (-225.5109, -596.7094) (-225.7735, -597.0801) (-226.0346, -597.4522) (-226.2943, -597.8258) (-226.5525, -598.2008) (-226.8094, -598.5772) (-227.0648, -598.955) (-227.3187, -599.3342) (-227.5713, -599.7148) (-227.8225, -600.0967) (-228.0723, -600.4799) (-228.3208, -600.8644) (-228.5678, -601.2503) (-228.8135, -601.6374) (-229.0579, -602.0258) (-229.3008, -602.4154) (-229.5425, -602.8064) (-229.7828, -603.1985) (-230.0218, -603.5919) (-230.2594, -603.9865) (-230.4957, -604.3822) (-230.7308, -604.7792) (-230.9645, -605.1773) (-231.1969, -605.5766) (-231.428, -605.9771) (-231.6578, -606.3787) (-231.8863, -606.7814) (-232.0681, -607.1045) (-232.2038, -607.3473) (-232.2941, -607.5094) (-232.3391, -607.5905) knots 0.10707295 0.10707295 0.10707295 0.10707295 0.10707295 0.10707295 0.11428571 0.12857143 0.14285714 0.15714286 0.17142857 0.18571429 0.2 0.21428571 0.22857143 0.24285714 0.25714286 0.27142857 0.28571429 0.3 0.31428571 0.32857143 0.34285714 0.35714286 0.37142857 0.38571429 0.4 0.41428571 0.42857143 0.44285714 0.45714286 0.47142857 0.48571429 0.5 0.51428571 0.52857143 0.54285714 0.55714286 0.57142857 0.58571429 0.6 0.61428571 0.62857143 0.64285714 0.65714286 0.67142857 0.68571429 0.7 0.71428571 0.72857143 0.74285714 0.75714286 0.77142857 0.78571429 0.8 0.81428571 0.82857143 0.84285714 0.85714286 0.87142857 0.88571429 0.9 0.91428571 0.92857143 0.94285714 0.95714286 0.97142857 0.98571429 1 1 1 1 1 1
  arc A11 (-232.3391, -607.5905) -> (-226.6005, -615.4891) centre (11.949, -436.1388) ccw
  spline S22 degree 5 poles (-226.6005, -615.4891) (-226.5094, -615.4713) (-226.3274, -615.4356) (-226.0545, -615.3815) (-225.691, -615.3084) (-225.2374, -615.2155) (-224.7844, -615.1211) (-224.3322, -615.025) (-223.8806, -614.9274) (-223.4297, -614.8282) (-222.9796, -614.7273) (-222.5302, -614.6249) (-222.0814, -614.5208) (-221.6335, -614.4151) (-221.1863, -614.3077) (-220.7398, -614.1987) (-220.2941, -614.088) (-219.8493, -613.9756) (-219.4051, -613.8616) (-218.9618, -613.7459) (-218.5194, -613.6284) (-218.0777, -613.5093) (-217.6369, -613.3884) (-217.1969, -613.2657) (-216.7578, -613.1414) (-216.3195, -613.0152) (-215.8822, -612.8873) (-215.4457, -612.7576) (-215.0102, -612.6261) (-214.5756, -612.4927) (-214.1419, -612.3575) (-213.7092, -612.2205) (-213.2774, -612.0816) (-212.8467, -611.9408) (-212.4169, -611.7981) (-211.9882, -611.6535) (-211.5605, -611.5069) (-211.1339, -611.3584) (-210.7084, -611.2079) (-210.284, -611.0554) (-209.8606, -610.9008) (-209.4385, -610.7442) (-209.0175, -610.5856) (-208.5976, -610.4248) (-208.179, -610.2619) (-207.7616, -610.0969) (-207.3455, -609.9296) (-206.9308, -609.7601) (-206.5173, -609.5883) (-206.1053, -609.4142) (-205.6946, -609.2377) (-205.2853, -609.0589) (-204.8775, -608.8778) (-204.4712, -608.6942) (-204.0664, -608.508) (-203.6632, -608.3192) (-203.2618, -608.1277) (-202.8622, -607.9334) (-202.4645, -607.7362) (-202.0686, -607.536) (-201.6746, -607.333) (-201.2825, -607.127) (-200.8923, -606.9181) (-200.5426, -606.7271) (-200.272, -606.5763) (-200.0794, -606.4673) (-199.9641, -606.4014) (-199.9254, -606.3792) knots -1 -1 -1 -1 -1 -1 -0.98571429 -0.97142857 -0.95714286 -0.94285714 -0.92857143 -0.91428571 -0.9 -0.88571429 -0.87142857 -0.85714286 -0.84285714 -0.82857143 -0.81428571 -0.8 -0.78571429 -0.77142857 -0.75714286 -0.74285714 -0.72857143 -0.71428571 -0.7 -0.68571429 -0.67142857 -0.65714286 -0.64285714 -0.62857143 -0.61428571 -0.6 -0.58571429 -0.57142857 -0.55714286 -0.54285714 -0.52857143 -0.51428571 -0.5 -0.48571429 -0.47142857 -0.45714286 -0.44285714 -0.42857143 -0.41428571 -0.4 -0.38571429 -0.37142857 -0.35714286 -0.34285714 -0.32857143 -0.31428571 -0.3 -0.28571429 -0.27142857 -0.25714286 -0.24285714 -0.22857143 -0.21428571 -0.2 -0.18571429 -0.17142857 -0.15714286 -0.14285714 -0.12857143 -0.11428571 -0.10707295 -0.10707295 -0.10707295 -0.10707295 -0.10707295 -0.10707295
  spline S23 degree 3 poles (-197.904, -606.755) (-198.0344, -606.5946) (-198.1949, -606.4612) (-198.558, -606.2634) (-198.7571, -606.201) (-199.1286, -606.1602) (-199.2964, -606.1683) (-199.6234, -606.2365) (-199.7805, -606.2962) (-199.9254, -606.3792) knots 0 0 0 0 0.062015 0.062015 0.12403 0.12403 0.174133 0.174133 0.224236 0.224236 0.224236 0.224236
  arc A12 (-197.904, -606.755) -> (-192.5158, -613.1764) centre (11.949, -436.1388) ccw
  spline S24 degree 3 poles (-192.4967, -615.2324) (-192.3643, -615.0736) (-192.2642, -614.8905) (-192.1398, -614.4963) (-192.1167, -614.2889) (-192.1479, -613.9164) (-192.188, -613.7533) (-192.3177, -613.4454) (-192.4064, -613.3027) (-192.5158, -613.1764) knots 0 0 0 0 0.062015 0.062015 0.12403 0.12403 0.174133 0.174133 0.224236 0.224236 0.224236 0.224236
  spline S25 degree 5 poles (-192.4967, -615.2324) (-192.5253, -615.2666) (-192.6102, -615.3688) (-192.751, -615.5395) (-192.9465, -615.7798) (-193.1953, -616.091) (-193.4688, -616.439) (-193.7397, -616.7894) (-194.0081, -617.1421) (-194.2739, -617.4972) (-194.5373, -617.8547) (-194.798, -618.2145) (-195.0563, -618.5765) (-195.3122, -618.9408) (-195.5659, -619.3071) (-195.8172, -619.6754) (-196.0665, -620.0455) (-196.3136, -620.4175) (-196.5587, -620.7914) (-196.8017, -621.1669) (-197.0427, -621.5442) (-197.2816, -621.9233) (-197.5186, -622.304) (-197.7537, -622.6864) (-197.9868, -623.0703) (-198.218, -623.4559) (-198.4473, -623.8429) (-198.6749, -624.2315) (-198.9006, -624.6216) (-199.1245, -625.0131) (-199.3466, -625.406) (-199.5669, -625.8003) (-199.7855, -626.1961) (-200.0024, -626.5932) (-200.2176, -626.9916) (-200.431, -627.3914) (-200.6428, -627.7924) (-200.8529, -628.1948) (-201.0613, -628.5984) (-201.2681, -629.0032) (-201.4733, -629.4093) (-201.6768, -629.8166) (-201.8787, -630.2251) (-202.079, -630.6348) (-202.2778, -631.0456) (-202.475, -631.4576) (-202.6706, -631.8708) (-202.8646, -632.285) (-203.0571, -632.7004) (-203.248, -633.1169) (-203.4375, -633.5344) (-203.6254, -633.9531) (-203.8118, -634.3727) (-203.9967, -634.7935) (-204.1801, -635.2153) (-204.362, -635.6381) (-204.5424, -636.0619) (-204.7213, -636.4867) (-204.8988, -636.9125) (-205.0748, -637.3393) (-205.2494, -637.767) (-205.4225, -638.1957) (-205.5942, -638.6254) (-205.7644, -639.056) (-205.8995, -639.4013) (-206.0001, -639.6606) (-206.0669, -639.8337) (-206.1003, -639.9203) knots 0.10707295 0.10707295 0.10707295 0.10707295 0.10707295 0.10707295 0.11428571 0.12857143 0.14285714 0.15714286 0.17142857 0.18571429 0.2 0.21428571 0.22857143 0.24285714 0.25714286 0.27142857 0.28571429 0.3 0.31428571 0.32857143 0.34285714 0.35714286 0.37142857 0.38571429 0.4 0.41428571 0.42857143 0.44285714 0.45714286 0.47142857 0.48571429 0.5 0.51428571 0.52857143 0.54285714 0.55714286 0.57142857 0.58571429 0.6 0.61428571 0.62857143 0.64285714 0.65714286 0.67142857 0.68571429 0.7 0.71428571 0.72857143 0.74285714 0.75714286 0.77142857 0.78571429 0.8 0.81428571 0.82857143 0.84285714 0.85714286 0.87142857 0.88571429 0.9 0.91428571 0.92857143 0.94285714 0.95714286 0.97142857 0.98571429 1 1 1 1 1 1
  arc A13 (-206.1003, -639.9203) -> (-199.3182, -646.9433) centre (11.949, -436.1388) ccw